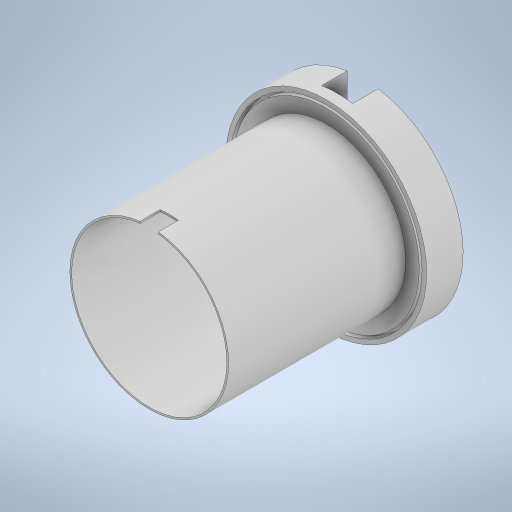
# Autodesk Inventor part: krabička
Saved by Autodesk Inventor 2024.2 (Build 282272000, 272)
## iProperties
Created: 2024-04-30
Part Number: krabička
Material: Všeobecné
Document SubType Name: Modeling
Designer: VÁCAL
Density: 1 g/cm^3
Appearance: Výchozí
Author: markoid
Autodesk Inventor part; units mm, degrees
ref_plane "YZ Plane" through (0, 0, 0) normal (1, 0, 0) x (0, 1, 0)
ref_plane "XZ Plane" through (0, 0, 0) normal (0, 1, 0) x (-1, 0, 0)
ref_plane "XY Plane" through (0, 0, 0) normal (0, 0, 1) x (1, 0, 0)
sketch "Náčrt1" plane through (0, 0, 0) normal (0, 0, 1) x (1, 0, 0)
  line L0 (0, 77) -> (0, -77) projected
  line L1 (-77, 0) -> (77, 0) projected
  circle A0 centre (0, 0) radius 55
  dimension "d0" = 110
  constraints: 1 centre point, 1 coincident
  measures "d0" diameter of A0
extrude "Vysunutí1" add sketch "Náčrt1" along normal blind 20
sketch "Náčrt3" plane through (0, 0, 20) normal (0, 0, 1) x (1, 0, 0)
  circle A0 centre (0, 0) radius 52.5
  circle A1 centre (0, 0) radius 51
  dimension "d7" = 105
  dimension "d8" = 102
  constraints: 2 centre point, 2 coincident
  measures "d7" diameter of A0
  measures "d8" diameter of A1
extrude "Vysunutí3" cut sketch "Náčrt3" against normal blind 3.5
sketch "Náčrt4" plane through (0, 0, 0) normal (0, 0, -1) x (-1, 0, 0)
  line L0 (-8.5, 55) -> (8.5, 55)
  line L1 (8.5, 55) -> (8.5, 15)
  line L2 (8.5, 15) -> (-8.5, 15)
  line L3 (-8.5, 15) -> (-8.5, 55)
  line L4 (0, -77) -> (0, 77) projected
  line L5 (-77, 0) -> (77, 0) projected
  circle A0 centre (0, 0) radius 55 projected
  point P0 (0, 55)
  dimension "d11" = 17
  dimension "d12" = 40
  constraints: 8 end point, 2 parallel, 1 horizontal, 1 midpoint, 1 perpendicular, 1 point on line, 1 vertical alignment, 1 other
  measures "d11" distance of L1.end L2.end
  measures "d12" distance of L0.end L1.end
extrude "Vysunutí4" cut sketch "Náčrt4" against normal blind 14 contours L0 A0 L3 | A0 L1 L2 L4 | L0 L1 A0 | L4 L2 L3 A0
sketch "Náčrt5" plane through (0, 0, 14) normal (0, 0, -1) x (-1, 0, 0)
  arc A0 (8.5, 54.3392) -> (-8.5, 54.3392) centre (0, 0) ccw projected
  line L0 (-8.5, 15) -> (-8.5, 54.3392) projected
  line L1 (8.5, 15) -> (-8.5, 15) projected
  line L2 (8.5, 54.3392) -> (8.5, 15) projected
  line L3 (-8.5, 15) -> (8.5, 15)
  line L4 (8.5, 15) -> (8.5, 22)
  line L5 (8.5, 22) -> (-8.5, 22)
  line L6 (-8.5, 22) -> (-8.5, 15)
  point P0 (-8.5, 22)
  dimension "d15" = 7
  constraints: 8 end point, 2 parallel, 1 horizontal, 1 perpendicular, 1 point on line
  measures "d15" distance of L4.end L3.end
extrude "Vysunutí5" cut sketch "Náčrt5" against normal through all contours L2 L1 L0 L5
sketch "Náčrt6" plane through (0, 0, 20) normal (0, 0, 1) x (1, 0, 0)
  circle A0 centre (0, 0) radius 43.5
  circle A1 centre (0, 0) radius 42.5
  line L0 (8.5, 15) -> (-8.5, 15) projected
  line L1 (-8.5, 15) -> (-8.5, 22) projected
  line L2 (-8.5, 22) -> (8.5, 22) projected
  line L3 (8.5, 22) -> (8.5, 15) projected
  circle A2 centre (0, 0) radius 51 projected
  line L4 (0, 77) -> (0, -77) projected
  dimension "d18" = 87
  dimension "d19" = 85
  constraints: 2 centre point, 2 coincident
  measures "d18" diameter of A0
  measures "d19" diameter of A1
extrude "Vysunutí6" add sketch "Náčrt6" along normal blind 97 contours A0 L4 A1 | L4 A1 A0
sketch "Náčrt7" plane through (0, 0, 117) normal (0, 0, 1) x (1, 0, 0)
  line L0 (5, 43.5) -> (-5, 43.5)
  line L1 (-5, 43.5) -> (-5, 33.5)
  line L2 (-5, 33.5) -> (5, 33.5)
  line L3 (5, 33.5) -> (5, 43.5)
  circle A0 centre (0, 0) radius 43.5 projected
  line L4 (0, 77) -> (0, -77) projected
  point P0 (0, 43.5)
  dimension "d22" = 10
  dimension "d23" = 10
  constraints: 8 end point, 2 parallel, 1 horizontal, 1 midpoint, 1 perpendicular, 1 point on line, 1 vertical alignment, 1 other
  measures "d22" distance of L2.end L1.end
  measures "d23" distance of L1.end L0.end
extrude "Vysunutí7" cut sketch "Náčrt7" against normal blind 11 contours L3 A0 L0 | A0 L1 L0 | L4 L2 L1 A0 | A0 L3 L2 L4 picked at (-2.7791, 36.7906) picked at (2.7791, 36.7906)
sketch "Náčrt8" plane through (0, 0, 20) normal (0, 0, 1) x (1, 0, 0)
  line L0 (7, -34.1663) -> (-7, -34.1663)
  line L1 (-7, -34.1663) -> (-7, -26.1663)
  line L2 (-7, -26.1663) -> (7, -26.1663)
  line L3 (7, -26.1663) -> (7, -34.1663)
  line L4 (0, 77) -> (0, -77) projected
  line L5 (-77, 0) -> (77, 0) projected
  line L6 (16.5, -39.1663) -> (-16.5, -39.1663)
  line L7 (-16.5, -39.1663) -> (-16.5, -34.1663)
  line L8 (-16.5, -34.1663) -> (16.5, -34.1663)
  line L9 (16.5, -34.1663) -> (16.5, -39.1663)
  arc A0 (-5, 42.2049) -> (5, 42.2049) centre (0, 0) ccw projected
  point P0 (0, -39.1663)
  point P1 (0, -34.1663)
  dimension "d26" = 33
  dimension "d27" = 5
  dimension "d28" = 14
  dimension "d29" = 8
  constraints: 16 end point, 4 parallel, 3 midpoint, 2 horizontal, 2 perpendicular, 2 point on line, 1 point on circle
  measures "d26" distance of L7.end L8.end
  measures "d27" distance of L6.end L7.end
  measures "d28" distance of L1.end L2.end
  measures "d29" distance of L0.end L1.end
extrude "Vysunutí8" add sketch "Náčrt8" along normal blind 32 contours L0 L4 L2 L3 | L0 L1 L2 L4
